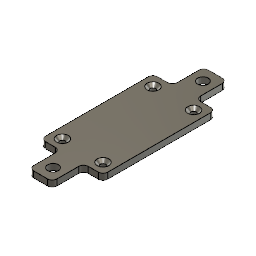
RPI PSU Bracket v1 (Autodesk Fusion 360 design; units mm, degrees)
Autodesk Fusion 360 part; units mm, degrees
sketch "Sketch1" plane through (0, 0, 0) normal (0, 1, 0) x (1, 0, 0)
  line L0 (13, 29) -> (-13, 29) construction
  line L1 (-13, 29) -> (-13, -29) construction
  line L2 (-13, -29) -> (13, -29) construction
  line L3 (13, -29) -> (13, 29) construction
  line L4 (13, 29) -> (-13, -29) construction
  line L5 (-13, 29) -> (13, -29) construction
  line L6 (0, 0) -> (0, 16.0365) construction
  line L7 (0, 0) -> (-11.1519, 0) construction
  line L8 (20, 36) -> (-20, 36)
  line L9 (-20, 36) -> (-20, -36)
  line L10 (-20, -36) -> (20, -36)
  line L11 (20, -36) -> (20, 36)
  line L12 (20, 36) -> (-20, -36) construction
  line L13 (-20, 36) -> (20, -36) construction
  circle A0 centre (13, 29) radius 1.75
  circle A1 centre (-13, 29) radius 1.75
  circle A2 centre (13, -29) radius 1.75
  circle A3 centre (-13, -29) radius 1.75
  line L14 (7.5, 36) -> (-7.5, 36)
  line L15 (-7.5, 36) -> (-7.5, 56)
  line L16 (-7.5, 56) -> (7.5, 56)
  line L17 (7.5, 56) -> (7.5, 36)
  line L18 (7.5, 36) -> (-7.5, 56) construction
  line L19 (-7.5, 36) -> (7.5, 56) construction
  circle A4 centre (0, 48) radius 3.4
  line L20 (7.5, -56) -> (7.5, -36)
  line L21 (-7.5, -56) -> (7.5, -56)
  line L22 (-7.5, -36) -> (-7.5, -56)
  circle A5 centre (0, -48) radius 3.4
  line L23 (7.5, -36) -> (-7.5, -36)
  point P0 (0, 46)
  dimension "d1" = 3.5
  dimension "d2" = 58
  dimension "d3" = 26
  dimension "d4" = 7
  dimension "d5" = 7
  dimension "d6" = 15
  dimension "d7" = 20
  dimension "d8" = 6.8
  dimension "d9" = 12
  constraint perpendicular L0 L1
  constraint parallel L0 L2
  constraint parallel L1 L3
  constraint horizontal L0
  constraint coincident L4 L6.start
  constraint coincident L5 L6.start
  constraint coincident L6.start L7.start
  constraint vertical L6
  constraint perpendicular L1 L7
  constraint perpendicular L8 L9
  constraint parallel L8 L10
  constraint parallel L9 L11
  constraint horizontal L8
  constraint coincident L12 L6.start
  constraint coincident L13 L6.start
  constraint coincident L0.start L3.end
  constraint symmetric L6 A0 A1
  constraint symmetric L7 A0 A2
  constraint symmetric L7 A1 A3
  constraint perpendicular L14 L15
  constraint parallel L14 L16
  constraint parallel L15 L17
  constraint horizontal L14
  constraint coincident L18 P0
  constraint coincident L19 P0
  constraint coincident L6 P0
  constraint coincident L8 L14.start
  constraint coincident L6 A4.centre
  constraint symmetric L7 L14.start L20.end
  constraint symmetric L7 L14.end L22.start
  constraint symmetric L7 L15.end L21.start
  constraint symmetric L7 L16.end L20.start
  constraint symmetric L7 A4 A5
  measures "d1" diameter of A0
  measures "d2" distance of L0.start L2.end
  measures "d3" distance of L0.start L0.end
  measures "d4" distance of L0 L8
  measures "d5" distance of L3 L11
  measures "d6" distance of L15.end L16.end
  measures "d7" distance of L14.start L16.end
  measures "d8" diameter of A4
  measures "d9" distance of L8 A4.centre
extrude "Extrude1" add sketch "Sketch1" along normal blind 4
fillet "Fillet1" radius 3 12 edges at (7.5, 2, 36) (20, 2, 36) (7.5, 2, 56) (-7.5, 2, 56) (-20, 2, 36) (-7.5, 2, 36) (20, 2, -36) (7.5, 2, -36) (7.5, 2, -56) (-7.5, 2, -56) (-20, 2, -36) (-7.5, 2, -36)
chamfer "Chamfer1" distance 2 angle 45 4 edges at (-14.6316, 4, -29.6328) (11.3684, 4, -29.6328) (11.3684, 4, 28.3672) (-14.6316, 4, 28.3672)
